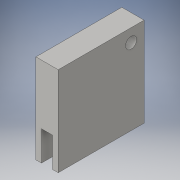
# Autodesk Inventor part: WideSupportForLift
Saved by Autodesk Inventor 2016 SP1 (Build 200210100, 210)
## iProperties
Created: 2016-02-14
Part Number: WideSupportForLift
Material: Generic
Document SubType Name: Modeling
Designer: steele
Density: 1 g/cm^3
Appearance: Default
Author: steele
Autodesk Inventor part; units mm, degrees
ref_plane "YZ Plane" through (0, 0, 0) normal (1, 0, 0) x (0, 1, 0)
ref_plane "XZ Plane" through (0, 0, 0) normal (0, 1, 0) x (-1, 0, 0)
ref_plane "XY Plane" through (0, 0, 0) normal (0, 0, 1) x (1, 0, 0)
sketch "Sketch6" plane through (0, 0, 0) normal (1, 0, 0) x (0, 1, 0)
  line L0 (-25.4, 36.6891) -> (-25.4, -36.6891)
  line L1 (-25.4, -36.6891) -> (0, -36.6891)
  line L2 (0, -36.6891) -> (0, 36.6891)
  line L3 (0, 36.6891) -> (-25.4, 36.6891)
  line L4 (-25.4, 36.6891) -> (0, -36.6891) construction
  line L5 (-25.4, -36.6891) -> (0, 36.6891) construction
  line L6 (0, 36.6891) -> (0, -36.6891)
  line L7 (0, -36.6891) -> (50.8, -36.6891)
  line L8 (50.8, -36.6891) -> (50.8, 36.6891)
  line L9 (50.8, 36.6891) -> (0, 36.6891)
  line L10 (0, 36.6891) -> (50.8, -36.6891) construction
  line L11 (0, -36.6891) -> (50.8, 36.6891) construction
  circle A0 centre (39.6875, -25.5766) radius 4.7625
  point P0 (0, 0)
  point P1 (-12.7, 0)
  point P2 (25.4, 0)
  dimension "d12" = 12.7
  dimension "d13" = 25.4
  dimension "d14" = 50.8
  dimension "d15" = 25.4
  dimension "d16" = 9.525
  dimension "d17" = 11.1125
  dimension "d18" = 11.1125
  constraints: 24 end point, 5 parallel, 4 midpoint, 2 perpendicular, 1 centre point, 1 vertical
  measures "d12" distance of point (-12.7, 0) point (0, 0)
  measures "d13" distance of point (0, 0) point (25.4, 0)
  measures "d14" distance of L8.end L6.start
  measures "d15" distance of L2.end L0.start
  measures "d16" diameter of A0
  measures "d17" distance from line of A0.centre L7
  measures "d18" distance from line of A0.centre L8
extrude "Extrusion3" add sketch "Sketch6" along normal mid plane 19.05
sketch "Sketch7" plane through (-9.525, -25.4, 36.6891) normal (0, 0, 1) x (1, 0, 0)
  line L0 (9.525, 25.4) -> (9.525, 0) construction
  line L1 (0, 0) -> (19.05, 0) construction
  line L2 (4.7625, 0) -> (14.2875, 0)
  line L3 (14.2875, 0) -> (14.2875, 25.4)
  line L4 (14.2875, 25.4) -> (4.7625, 25.4)
  line L5 (4.7625, 25.4) -> (4.7625, 0)
  line L6 (4.7625, 0) -> (14.2875, 25.4) construction
  line L7 (14.2875, 0) -> (4.7625, 25.4) construction
  point P0 (9.525, 12.7)
  dimension "d21" = 9.525
  constraints: 14 end point, 4 midpoint, 2 parallel, 1 horizontal, 1 perpendicular
  measures "d21" distance between parallel lines of L3 L5
extrude "Extrusion4" cut sketch "Sketch7" against normal through all
body "Solid2"
